Autodesk Inventor part; units mm, degrees
(part 3 of 3)
  arc A561 (-5.9494, 3.2712) -> (-5.9494, -2.9864) centre (0.0316, 0.1424) ccw projected
  arc A562 (-5.9494, 3.2712) -> (-5.9494, -2.9864) centre (0.0316, 0.1424) ccw projected
  arc A563 (-5.9494, 3.2712) -> (-5.9494, -2.9864) centre (0.0316, 0.1424) ccw projected
  arc A564 (-5.9494, 3.2712) -> (-5.9494, -2.9864) centre (0.0316, 0.1424) ccw projected
  arc A565 (-5.9494, 3.2712) -> (-5.9494, -2.9864) centre (0.0316, 0.1424) ccw projected
  arc A566 (-5.9494, 3.2712) -> (-5.9494, -2.9864) centre (0.0316, 0.1424) ccw projected
  circle A567 centre (0.0316, 0.1424) radius 2.5 projected
  circle A568 centre (0.0316, 0.1424) radius 2.5 projected
  circle A569 centre (0.0316, 0.1424) radius 2.5 projected
  circle A570 centre (0.0316, 0.1424) radius 2.5 projected
  circle A571 centre (0.0316, 0.1424) radius 5.5 projected
  circle A572 centre (0.0316, 0.1424) radius 6.75 projected
  arc A573 (3.1605, 6.1234) -> (-3.0972, 6.1234) centre (0.0316, 0.1424) ccw projected
  arc A574 (3.1605, 6.1234) -> (-3.0972, 6.1234) centre (0.0316, 0.1424) ccw projected
  arc A575 (3.1605, 6.1234) -> (-3.0972, 6.1234) centre (0.0316, 0.1424) ccw projected
  arc A576 (3.1605, 6.1234) -> (-3.0972, 6.1234) centre (0.0316, 0.1424) ccw projected
  arc A577 (3.1605, 6.1234) -> (-3.0972, 6.1234) centre (0.0316, 0.1424) ccw projected
  arc A578 (3.1605, 6.1234) -> (-3.0972, 6.1234) centre (0.0316, 0.1424) ccw projected
  arc A579 (6.0127, -2.9864) -> (6.0127, 3.2712) centre (0.0316, 0.1424) ccw projected
  arc A580 (6.0127, -2.9864) -> (6.0127, 3.2712) centre (0.0316, 0.1424) ccw projected
  arc A581 (6.0127, -2.9864) -> (6.0127, 3.2712) centre (0.0316, 0.1424) ccw projected
  arc A582 (6.0127, -2.9864) -> (6.0127, 3.2712) centre (0.0316, 0.1424) ccw projected
  arc A583 (6.0127, -2.9864) -> (6.0127, 3.2712) centre (0.0316, 0.1424) ccw projected
  arc A584 (6.0127, -2.9864) -> (6.0127, 3.2712) centre (0.0316, 0.1424) ccw projected
  line L286 (0.0316, 0.1424) -> (12.7316, 0.1424) projected
  line L287 (0.0316, 0.1424) -> (12.7316, 0.1424) projected
  line L288 (3.1605, 12.915) -> (3.1605, 6.1234) projected
  line L289 (3.1605, 12.915) -> (3.1605, 6.1234) projected
  line L290 (0.0316, 0.1424) -> (0.0316, 12.8424) projected
  line L291 (0.0316, 0.1424) -> (0.0316, 12.8424) projected
  circle A585 centre (8.6605, 19.3778) radius 1.5 projected
  line L292 (6.1605, 19.3778) -> (3.1605, 19.3778) projected
  arc A586 (4.7714, 23.2669) -> (3.1605, 19.3778) centre (8.6605, 19.3778) ccw projected
  arc A587 (4.7714, 23.2669) -> (3.1605, 19.3778) centre (8.6605, 19.3778) ccw projected
  arc A588 (4.7714, 23.2669) -> (3.1605, 19.3778) centre (8.6605, 19.3778) ccw projected
  circle A589 centre (8.6605, 19.3778) radius 2.5 projected
  circle A590 centre (8.6605, 19.3778) radius 2.5 projected
  circle A591 centre (8.6605, 19.3778) radius 3 projected
  arc A592 (3.1605, 19.3778) -> (4.7714, 23.2669) centre (8.6605, 19.3778) ccw projected
  arc A593 (3.1605, 19.3778) -> (4.7714, 23.2669) centre (8.6605, 19.3778) ccw projected
  circle A594 centre (8.6605, 19.3778) radius 5.5 projected
  circle A595 centre (8.6605, 19.3778) radius 5.5 projected
  circle A596 centre (8.6605, 19.3778) radius 5.5 projected
  circle A597 centre (8.6605, 19.3778) radius 5.5 projected
  arc A598 (3.1605, 19.3778) -> (4.7714, 23.2669) centre (8.6605, 19.3778) ccw projected
  line L293 (6.0127, 3.2712) -> (19.2671, 3.2712) projected
  line L294 (6.0127, 3.2712) -> (19.2671, 3.2712) projected
  line L295 (6.0127, 3.2712) -> (19.2671, 3.2712) projected
  line L296 (19.2671, 3.2712) -> (6.0127, 3.2712) projected
  line L297 (6.0127, 3.2712) -> (19.2671, 3.2712) projected
  line L298 (6.0127, 3.2712) -> (19.2671, 3.2712) projected
  line L299 (6.0127, 3.2712) -> (19.2671, 3.2712) projected
  line L300 (22.4784, 40.9739) -> (4.7714, 23.2669) projected
  line L301 (22.4784, 40.9739) -> (4.7714, 23.2669) projected
  line L302 (13.2567, 31.7522) -> (4.7714, 23.2669) projected
  line L303 (13.2567, 31.7522) -> (4.7714, 23.2669) projected
  line L304 (22.4784, 40.9739) -> (13.2567, 31.7522) projected
  line L305 (13.2567, 31.7522) -> (4.7714, 23.2669) projected
  line L306 (22.4784, 40.9739) -> (4.7714, 23.2669) projected
  line L307 (13.2567, 31.7522) -> (4.7714, 23.2669) projected
  circle A599 centre (17.1458, 27.8631) radius 1.5 projected
  circle A600 centre (17.1458, 27.8631) radius 3 projected
  circle A601 centre (17.1458, 27.8631) radius 2.5 projected
  circle A602 centre (17.1458, 27.8631) radius 2.5 projected
  circle A603 centre (17.1458, 27.8631) radius 5.5 projected
  circle A604 centre (17.1458, 27.8631) radius 5.5 projected
  circle A605 centre (17.1458, 27.8631) radius 5.5 projected
  circle A606 centre (17.1458, 27.8631) radius 5.5 projected
  circle A607 centre (17.1458, 27.8631) radius 5.5 projected
  circle A608 centre (17.1458, 27.8631) radius 5.5 projected
  circle A609 centre (17.1458, 27.8631) radius 5.5 projected
  arc A610 (19.2671, 3.2712) -> (23.1562, 4.8822) centre (19.2671, 8.7712) ccw projected
  arc A611 (19.2671, 3.2712) -> (23.1562, 4.8822) centre (19.2671, 8.7712) ccw projected
  arc A612 (19.2671, 3.2712) -> (23.1562, 4.8822) centre (19.2671, 8.7712) ccw projected
  circle A613 centre (19.2671, 8.7712) radius 1.5 projected
  circle A614 centre (19.2671, 8.7712) radius 2.5 projected
  circle A615 centre (19.2671, 8.7712) radius 2.5 projected
  circle A616 centre (19.2671, 8.7712) radius 3 projected
  arc A617 (23.1562, 4.8822) -> (19.2671, 3.2712) centre (19.2671, 8.7712) ccw projected
  arc A618 (23.1562, 4.8822) -> (19.2671, 3.2712) centre (19.2671, 8.7712) ccw projected
  circle A619 centre (19.2671, 8.7712) radius 5.5 projected
  circle A620 centre (19.2671, 8.7712) radius 5.5 projected
  circle A621 centre (19.2671, 8.7712) radius 5.5 projected
  arc A622 (23.1562, 4.8822) -> (19.2671, 3.2712) centre (19.2671, 8.7712) ccw projected
  circle A623 centre (19.2671, 8.7712) radius 5.5 projected
  arc A624 (14.3956, 11.3243) -> (23.1562, 4.8822) centre (19.2671, 8.7712) ccw projected
  line L308 (23.1562, 4.8822) -> (31.6415, 13.3674) projected
  line L309 (23.1562, 4.8822) -> (31.6415, 13.3674) projected
  line L310 (23.1562, 4.8822) -> (31.6415, 13.3674) projected
  line L311 (31.6415, 13.3674) -> (23.1562, 4.8822) projected
  line L312 (22.4784, 40.9739) -> (13.2567, 31.7522) projected
  line L313 (22.4784, 40.9739) -> (13.2567, 31.7522) projected
  line L314 (13.2567, 31.7522) -> (22.4784, 40.9739) projected
  line L315 (33.6153, 29.837) -> (29.7263, 33.7261) projected
  line L316 (29.7263, 33.7261) -> (22.4784, 40.9739) projected
  line L317 (40.8632, 22.5892) -> (22.4784, 40.9739) projected
  line L318 (40.8632, 22.5892) -> (22.4784, 40.9739) projected
  line L319 (40.8632, 22.5892) -> (22.4784, 40.9739) projected
  line L320 (40.8632, 22.5892) -> (22.4784, 40.9739) projected
  line L321 (40.8632, 22.5892) -> (22.4784, 40.9739) projected
  line L322 (40.8632, 22.5892) -> (22.4784, 40.9739) projected
  line L323 (33.6153, 29.837) -> (40.8632, 22.5892) projected
  line L324 (31.6415, 13.3674) -> (40.8632, 22.5892) projected
  circle A625 centre (27.7524, 17.2565) radius 1.5 projected
  circle A626 centre (27.7524, 17.2565) radius 2.5 projected
  circle A627 centre (27.7524, 17.2565) radius 2.5 projected
  circle A628 centre (27.7524, 17.2565) radius 3 projected
  circle A629 centre (27.7524, 17.2565) radius 5.5 projected
  circle A630 centre (27.7524, 17.2565) radius 5.5 projected
  circle A631 centre (27.7524, 17.2565) radius 5.5 projected
  circle A632 centre (27.7524, 17.2565) radius 5.5 projected
  circle A633 centre (27.7524, 17.2565) radius 5.5 projected
  circle A634 centre (27.7524, 17.2565) radius 5.5 projected
  circle A635 centre (27.7524, 17.2565) radius 5.5 projected
  line L325 (23.1562, 4.8822) -> (40.8632, 22.5892) projected
  line L326 (23.1562, 4.8822) -> (40.8632, 22.5892) projected
  line L327 (23.1562, 4.8822) -> (40.8632, 22.5892) projected
  line L328 (31.6415, 13.3674) -> (40.8632, 22.5892) projected
  line L329 (31.6415, 13.3674) -> (40.8632, 22.5892) projected
  line L330 (31.6415, 13.3674) -> (40.8632, 22.5892) projected
  line L331 (-13.1934, -31.4674) -> (-22.4151, -40.6891) projected
  line L332 (-22.4151, -40.6891) -> (-13.1934, -31.4674) projected
  line L333 (-22.4151, -40.6891) -> (-13.1934, -31.4674) projected
  line L334 (-22.4151, -40.6891) -> (-13.1934, -31.4674) projected
  line L335 (-22.4151, -40.6891) -> (-4.7081, -22.9821) projected
  line L336 (-22.4151, -40.6891) -> (-4.7081, -22.9821) projected
  line L337 (-22.4151, -40.6891) -> (-4.7081, -22.9821) projected
  circle A636 centre (-17.0825, -27.5783) radius 1.5 projected
  circle A637 centre (-17.0825, -27.5783) radius 2.5 projected
  circle A638 centre (-17.0825, -27.5783) radius 2.5 projected
  circle A639 centre (-17.0825, -27.5783) radius 5.5 projected
  circle A640 centre (-17.0825, -27.5783) radius 5.5 projected
  circle A641 centre (-17.0825, -27.5783) radius 5.5 projected
  circle A642 centre (-17.0825, -27.5783) radius 5.5 projected
  circle A643 centre (-17.0825, -27.5783) radius 5.5 projected
  circle A644 centre (-17.0825, -27.5783) radius 5.5 projected
  circle A645 centre (-17.0825, -27.5783) radius 5.5 projected
  line L338 (6.1605, -19.0931) -> (3.1605, -19.0931) projected
  arc A646 (3.1605, -19.0931) -> (4.7714, -22.9821) centre (8.6605, -19.0931) ccw projected
  arc A647 (3.1605, -19.0931) -> (4.7714, -22.9821) centre (8.6605, -19.0931) ccw projected
  arc A648 (3.1605, -19.0931) -> (4.7714, -22.9821) centre (8.6605, -19.0931) ccw projected
  line L339 (3.1605, -19.0931) -> (3.1605, -12.6302) projected
  line L340 (3.1605, -19.0931) -> (3.1605, -12.6302) projected
  line L341 (14.3226, -10.9666) -> (14.3956, -11.0396) projected
  circle A649 centre (19.2671, -8.4864) radius 1.5 projected
  circle A650 centre (19.2671, -8.4864) radius 2.5 projected
  circle A651 centre (19.2671, -8.4864) radius 2.5 projected
  circle A652 centre (19.2671, -8.4864) radius 2.5 projected
  circle A653 centre (19.2671, -8.4864) radius 2.5 projected
  arc A654 (23.1562, -4.5974) -> (14.3956, -11.0396) centre (19.2671, -8.4864) ccw projected
  line L342 (17.4993, -10.2542) -> (23.1562, -4.5974) projected
  arc A655 (23.1562, -4.5974) -> (14.3956, -11.0396) centre (19.2671, -8.4864) ccw projected
  line L343 (-5.9494, -2.9864) -> (-19.2038, -2.9864) projected
  line L344 (-5.9494, -2.9864) -> (-19.2038, -2.9864) projected
  line L345 (-5.9494, -2.9864) -> (-19.2038, -2.9864) projected
  line L346 (-5.9494, -2.9864) -> (-19.2038, -2.9864) projected
  line L347 (-5.9494, -2.9864) -> (-19.2038, -2.9864) projected
  line L348 (-5.9494, -2.9864) -> (-19.2038, -2.9864) projected
  line L349 (-19.2038, -2.9864) -> (-5.9494, -2.9864) projected
  arc A656 (4.7714, -22.9821) -> (3.1605, -19.0931) centre (8.6605, -19.0931) ccw projected
  arc A657 (4.7714, -22.9821) -> (3.1605, -19.0931) centre (8.6605, -19.0931) ccw projected
  circle A658 centre (8.6605, -19.0931) radius 5.5 projected
  circle A659 centre (8.6605, -19.0931) radius 5.5 projected
  arc A660 (4.7714, -22.9821) -> (3.1605, -19.0931) centre (8.6605, -19.0931) ccw projected
  circle A661 centre (8.6605, -19.0931) radius 5.5 projected
  circle A662 centre (8.6605, -19.0931) radius 5.5 projected
  circle A663 centre (8.6605, -19.0931) radius 5.5 projected
  circle A664 centre (8.6605, -19.0931) radius 2.5 projected
  circle A665 centre (8.6605, -19.0931) radius 2.5 projected
  circle A666 centre (8.6605, -19.0931) radius 2.5 projected
  circle A667 centre (8.6605, -19.0931) radius 1.5 projected
  line L350 (-23.0929, -4.5974) -> (-40.7999, -22.3044) projected
  circle A668 centre (-27.6891, -16.9717) radius 1.5 projected
  circle A669 centre (-27.6891, -16.9717) radius 2.5 projected
  circle A670 centre (-27.6891, -16.9717) radius 2.5 projected
  line L351 (-23.0929, -4.5974) -> (-40.7999, -22.3044) projected
  line L352 (-23.0929, -4.5974) -> (-40.7999, -22.3044) projected
  line L353 (-31.5782, -13.0826) -> (-40.7999, -22.3044) projected
  circle A671 centre (-27.6891, -16.9717) radius 5.5 projected
  circle A672 centre (-27.6891, -16.9717) radius 5.5 projected
  circle A673 centre (-27.6891, -16.9717) radius 5.5 projected
  circle A674 centre (-27.6891, -16.9717) radius 5.5 projected
  circle A675 centre (-27.6891, -16.9717) radius 5.5 projected
  circle A676 centre (-27.6891, -16.9717) radius 5.5 projected
  circle A677 centre (-27.6891, -16.9717) radius 5.5 projected
  line L354 (-6.9395, -3.6467) -> (-6.2792, -2.9864) projected
  line L355 (0.0316, 0.1424) -> (-12.6684, 0.1424) projected
  line L356 (0.0316, 0.1424) -> (-12.6684, 0.1424) projected
  line L357 (0.0316, 0.1424) -> (0.0316, -12.5576) projected
  line L358 (-23.0929, -4.5974) -> (-31.5782, -13.0826) projected
  line L359 (-23.0929, -4.5974) -> (-31.5782, -13.0826) projected
  line L360 (-23.0929, -4.5974) -> (-31.5782, -13.0826) projected
  arc A678 (-19.2038, -2.9864) -> (-23.0929, -4.5974) centre (-19.2038, -8.4864) ccw projected
  arc A679 (-23.0929, -4.5974) -> (-19.2038, -2.9864) centre (-19.2038, -8.4864) ccw projected
  arc A680 (-19.2038, -2.9864) -> (-23.0929, -4.5974) centre (-19.2038, -8.4864) ccw projected
  arc A681 (-23.0929, -4.5974) -> (-19.2038, -2.9864) centre (-19.2038, -8.4864) ccw projected
  circle A682 centre (-19.2038, -8.4864) radius 5.5 projected
  circle A683 centre (-19.2038, -8.4864) radius 5.5 projected
  arc A684 (-19.2038, -2.9864) -> (-23.0929, -4.5974) centre (-19.2038, -8.4864) ccw projected
  arc A685 (-23.0929, -4.5974) -> (-19.2038, -2.9864) centre (-19.2038, -8.4864) ccw projected
  circle A686 centre (-19.2038, -8.4864) radius 5.5 projected
  line L361 (-31.5782, -13.0826) -> (-23.0929, -4.5974) projected
  circle A687 centre (-19.2038, -8.4864) radius 2.5 projected
  circle A688 centre (-19.2038, -8.4864) radius 2.5 projected
  circle A689 centre (-19.2038, -8.4864) radius 5.5 projected
  arc A690 (-14.3323, -11.0396) -> (-23.0929, -4.5974) centre (-19.2038, -8.4864) ccw projected
  arc A691 (-14.3323, -11.0396) -> (-23.0929, -4.5974) centre (-19.2038, -8.4864) ccw projected
  circle A692 centre (-19.2038, -8.4864) radius 1.5 projected
  arc A693 (-3.0972, -5.8386) -> (3.1605, -5.8386) centre (0.0316, 0.1424) ccw projected
  arc A694 (-3.0972, -5.8386) -> (3.1605, -5.8386) centre (0.0316, 0.1424) ccw projected
  arc A695 (-3.0972, -5.8386) -> (3.1605, -5.8386) centre (0.0316, 0.1424) ccw projected
  arc A696 (-3.0972, -5.8386) -> (3.1605, -5.8386) centre (0.0316, 0.1424) ccw projected
  arc A697 (-3.0972, -5.8386) -> (3.1605, -5.8386) centre (0.0316, 0.1424) ccw projected
  arc A698 (-3.0972, -5.8386) -> (3.1605, -5.8386) centre (0.0316, 0.1424) ccw projected
  line L362 (3.1605, -12.6302) -> (3.1605, -5.8386) projected
  line L363 (3.1605, -12.6302) -> (3.1605, -5.8386) projected
  line L364 (-3.0972, -12.6302) -> (-3.0972, -5.8386) projected
  line L365 (-3.0972, -12.6302) -> (-3.0972, -5.8386) projected
  circle A699 centre (0.0316, -12.5576) radius 2.5 projected
  circle A700 centre (0.0316, -12.5576) radius 2.5 projected
  line L366 (3.1605, -5.8386) -> (3.1605, -19.0931) projected
  line L367 (-3.0972, -19.0931) -> (-3.0972, -5.8386) projected
  line L368 (-3.0972, -19.0931) -> (-3.0972, -5.8386) projected
  line L369 (-3.0972, -19.0931) -> (-3.0972, -5.8386) projected
  line L370 (-3.0972, -19.0931) -> (-3.0972, -5.8386) projected
  line L371 (-3.0972, -19.0931) -> (-3.0972, -5.8386) projected
  line L372 (-3.0972, -19.0931) -> (-3.0972, -5.8386) projected
  line L373 (3.1605, -5.8386) -> (3.1605, -19.0931) projected
  line L374 (3.1605, -5.8386) -> (3.1605, -19.0931) projected
  line L375 (3.1605, -5.8386) -> (3.1605, -19.0931) projected
  line L376 (3.1605, -5.8386) -> (3.1605, -19.0931) projected
  line L377 (3.1605, -5.8386) -> (3.1605, -19.0931) projected
  line L378 (-6.0972, -19.0931) -> (-3.0972, -19.0931) projected
  line L379 (-3.0972, -19.0931) -> (-3.0972, -12.6302) projected
  line L380 (-3.0972, -19.0931) -> (-3.0972, -12.6302) projected
  line L381 (-31.5782, -13.0826) -> (-40.7999, -22.3044) projected
  line L382 (-31.5782, -13.0826) -> (-40.7999, -22.3044) projected
  line L383 (-31.5782, -13.0826) -> (-40.7999, -22.3044) projected
  line L384 (-40.7999, -22.3044) -> (-22.4151, -40.6891) projected
  line L385 (-40.7999, -22.3044) -> (-22.4151, -40.6891) projected
  line L386 (-40.7999, -22.3044) -> (-22.4151, -40.6891) projected
  line L387 (-40.7999, -22.3044) -> (-22.4151, -40.6891) projected
  line L388 (-33.5521, -29.5522) -> (-40.7999, -22.3044) projected
  line L389 (-33.5521, -29.5522) -> (-29.663, -33.4413) projected
  line L390 (-29.663, -33.4413) -> (-22.4151, -40.6891) projected
  line L391 (-40.7999, -22.3044) -> (-22.4151, -40.6891) projected
  line L392 (-40.7999, -22.3044) -> (-22.4151, -40.6891) projected
  arc A701 (-4.7081, -22.9821) -> (-3.0972, -19.0931) centre (-8.5972, -19.0931) ccw projected
  arc A702 (-3.0972, -19.0931) -> (-4.7081, -22.9821) centre (-8.5972, -19.0931) ccw projected
  line L393 (-13.1934, -31.4674) -> (-4.7081, -22.9821) projected
  arc A703 (-4.7081, -22.9821) -> (-3.0972, -19.0931) centre (-8.5972, -19.0931) ccw projected
  line L394 (-13.1934, -31.4674) -> (-4.7081, -22.9821) projected
  arc A704 (-3.0972, -19.0931) -> (-4.7081, -22.9821) centre (-8.5972, -19.0931) ccw projected
  circle A705 centre (-8.5972, -19.0931) radius 5.5 projected
  circle A706 centre (-8.5972, -19.0931) radius 5.5 projected
  circle A707 centre (-8.5972, -19.0931) radius 1.5 projected
  circle A708 centre (-8.5972, -19.0931) radius 2.5 projected
  circle A709 centre (-8.5972, -19.0931) radius 2.5 projected
  circle A710 centre (-8.5972, -19.0931) radius 5.5 projected
  arc A711 (-3.0972, -19.0931) -> (-4.7081, -22.9821) centre (-8.5972, -19.0931) ccw projected
  circle A712 centre (-8.5972, -19.0931) radius 5.5 projected
  arc A713 (-4.7081, -22.9821) -> (-3.0972, -19.0931) centre (-8.5972, -19.0931) ccw projected
  line L395 (-13.1934, -31.4674) -> (-4.7081, -22.9821) projected
  line L396 (-13.1934, -31.4674) -> (-4.7081, -22.9821) projected
  line L397 (12.7316, -10.3076) -> (12.7316, -12.5576) projected
  line L398 (12.7316, -10.3076) -> (12.7316, -12.5576) projected
  line L399 (12.7316, -10.3076) -> (12.7316, -12.5576) projected
  line L400 (12.7316, -12.5576) -> (10.4816, -12.5576) projected
  line L401 (12.7316, -12.5576) -> (10.4816, -12.5576) projected
  line L402 (12.7316, -12.5576) -> (10.4816, -12.5576) projected
  arc A714 (10.4816, -12.5576) -> (11.1407, -14.1486) centre (12.7316, -12.5576) ccw projected
  arc A715 (10.4816, -12.5576) -> (11.1407, -14.1486) centre (12.7316, -12.5576) ccw projected
  arc A716 (10.4816, -12.5576) -> (11.1407, -14.1486) centre (12.7316, -12.5576) ccw projected
  arc A717 (10.5886, -13.2429) -> (11.1407, -14.1486) centre (12.7316, -12.5576) ccw projected
  arc A718 (10.5886, -13.2429) -> (11.1407, -14.1486) centre (12.7316, -12.5576) ccw projected
  arc A719 (23.1562, -4.5974) -> (19.2671, -2.9864) centre (19.2671, -8.4864) ccw projected
  arc A720 (23.1562, -4.5974) -> (19.2671, -2.9864) centre (19.2671, -8.4864) ccw projected
  arc A721 (23.1562, -4.5974) -> (19.2671, -2.9864) centre (19.2671, -8.4864) ccw projected
  arc A722 (23.1562, -4.5974) -> (14.3956, -11.0396) centre (19.2671, -8.4864) ccw projected
  line L403 (15.378, -12.3755) -> (15.9083, -11.8452) projected
  line L404 (15.5548, -12.1988) -> (15.9136, -12.5576) projected
  arc A723 (15.378, -12.3755) -> (15.569, -12.5576) centre (19.2671, -8.4864) ccw projected
  arc A724 (15.378, -12.3755) -> (15.569, -12.5576) centre (19.2671, -8.4864) ccw projected
  arc A725 (19.2671, -2.9864) -> (23.1562, -4.5974) centre (19.2671, -8.4864) ccw projected
  arc A726 (19.2671, -2.9864) -> (23.1562, -4.5974) centre (19.2671, -8.4864) ccw projected
  circle A727 centre (19.2671, -8.4864) radius 5.5 projected
  arc A728 (19.2671, -2.9864) -> (23.1562, -4.5974) centre (19.2671, -8.4864) ccw projected
  circle A729 centre (19.2671, -8.4864) radius 5.5 projected
  circle A730 centre (19.2671, -8.4864) radius 5.5 projected
  circle A731 centre (19.2671, -8.4864) radius 5.5 projected
  line L405 (17.5046, -14.1486) -> (14.3226, -10.9666) projected
  line L406 (24.3936, -20.3305) -> (16.8521, -20.3305) construction
  line L407 (17.5046, -14.1486) -> (26.1667, -22.8107) projected
  line L408 (26.1667, -22.8107) -> (14.3226, -10.9666) projected
  line L409 (14.3226, -10.9666) -> (26.1667, -22.8107) projected
  line L410 (26.1667, -22.8107) -> (14.3226, -10.9666) projected
  arc A732 (14.3226, -17.3306) -> (18.0567, -15.0542) centre (15.9136, -15.7396) ccw projected
  arc A733 (14.3226, -17.3306) -> (17.5046, -14.1486) centre (15.9136, -15.7396) ccw projected
  arc A734 (14.3226, -17.3306) -> (17.5046, -14.1486) centre (15.9136, -15.7396) ccw projected
  line L411 (20.5045, -20.3305) -> (23.3382, -23.1642) projected
  line L412 (20.5045, -20.3305) -> (23.3382, -23.1642) projected
  line L413 (20.5045, -24.2196) -> (13.9798, -17.6948) projected
  line L414 (12.3728, -15.3807) -> (12.5496, -15.204) projected
  line L415 (22.9847, -25.9926) -> (14.3226, -17.3306) projected
  line L416 (11.1407, -14.1486) -> (12.3728, -15.3807) projected
  line L417 (11.1407, -14.1486) -> (14.3226, -17.3306) projected
  line L418 (11.1407, -14.1486) -> (22.9847, -25.9926) projected
  line L419 (11.1407, -14.1486) -> (22.9847, -25.9926) projected
  line L420 (22.9847, -25.9926) -> (11.1407, -14.1486) projected
  line L421 (23.1615, -25.8159) -> (10.5886, -13.2429) projected
  line L422 (23.1615, -25.8159) -> (10.5886, -13.2429) projected
  line L423 (25.9899, -22.9874) -> (13.417, -10.4145) projected
  line L424 (40.8632, -22.3044) -> (23.1562, -4.5974) projected
  line L425 (40.8632, -22.3044) -> (23.1562, -4.5974) projected
  line L426 (31.6415, -13.0826) -> (23.1562, -4.5974) projected
  line L427 (31.6415, -13.0826) -> (23.1562, -4.5974) projected
  line L428 (31.6415, -13.0826) -> (23.1562, -4.5974) projected
  line L429 (31.6415, -13.0826) -> (23.1562, -4.5974) projected
  line L430 (31.6415, -13.0826) -> (23.1562, -4.5974) projected
  arc A735 (31.6415, -13.0826) -> (22.4331, -18.3699) centre (27.7524, -16.9717) ccw projected
  line L431 (22.4331, -18.3699) -> (26.3542, -22.291) projected
  line L432 (40.8632, -22.3044) -> (23.1562, -4.5974) projected
  arc A736 (26.3542, -22.291) -> (31.6415, -13.0826) centre (27.7524, -16.9717) ccw projected
  line L433 (40.8632, -22.3044) -> (31.6415, -13.0826) projected
  line L434 (4.7714, -22.9821) -> (22.4784, -40.6891) projected
  line L435 (22.4784, -40.6891) -> (40.8632, -22.3044) projected
  line L436 (4.7714, -22.9821) -> (22.4784, -40.6891) projected
  line L437 (22.4784, -40.6891) -> (40.8632, -22.3044) projected
  line L438 (22.4784, -40.6891) -> (40.8632, -22.3044) projected
  line L439 (13.2567, -31.4674) -> (22.4784, -40.6891) projected
  arc A737 (13.2567, -31.4674) -> (22.4651, -26.1801) centre (17.1458, -27.5783) ccw projected
  line L440 (22.4651, -26.1801) -> (18.544, -22.259) projected
  arc A738 (18.544, -22.259) -> (13.2567, -31.4674) centre (17.1458, -27.5783) ccw projected
  line L441 (4.7714, -22.9821) -> (13.2567, -31.4674) projected
  line L442 (4.7714, -22.9821) -> (13.2567, -31.4674) projected
  line L443 (4.7714, -22.9821) -> (13.2567, -31.4674) projected
  line L444 (13.2567, -31.4674) -> (4.7714, -22.9821) projected
  line L445 (13.2567, -31.4674) -> (4.7714, -22.9821) projected
  line L446 (4.7714, -22.9821) -> (22.4784, -40.6891) projected
  line L447 (19.2671, -2.9864) -> (6.0127, -2.9864) projected
  line L448 (19.2671, -2.9864) -> (6.0127, -2.9864) projected
  line L449 (19.2671, -2.9864) -> (6.0127, -2.9864) projected
  line L450 (19.2671, -2.9864) -> (6.0127, -2.9864) projected
  line L451 (19.2671, -2.9864) -> (6.0127, -2.9864) projected
  line L452 (19.2671, -2.9864) -> (6.0127, -2.9864) projected
  arc A739 (14.3226, -10.9666) -> (13.417, -10.4145) centre (12.7316, -12.5576) ccw projected
  arc A740 (14.3226, -10.9666) -> (13.417, -10.4145) centre (12.7316, -12.5576) ccw projected
  arc A741 (14.3226, -10.9666) -> (12.7316, -10.3076) centre (12.7316, -12.5576) ccw projected
  arc A742 (14.3226, -10.9666) -> (12.7316, -10.3076) centre (12.7316, -12.5576) ccw projected
  arc A743 (14.3226, -10.9666) -> (12.7316, -10.3076) centre (12.7316, -12.5576) ccw projected
  line L453 (7.0028, -3.6467) -> (6.3425, -2.9864) projected
  line L454 (19.2671, -2.9864) -> (6.0127, -2.9864) projected
  line L455 (19.2671, -2.9864) -> (6.0127, -2.9864) projected
  line L456 (14.3226, -10.9666) -> (7.0028, -3.6467) projected
  line L457 (14.3226, -10.9666) -> (3.9708, -10.9666) construction
  line L458 (25.9899, -22.9874) -> (26.1667, -22.8107) projected
  line L459 (26.1667, -22.8107) -> (25.9899, -22.9874) projected
  line L460 (29.7263, -25.6631) -> (33.6153, -29.5522) projected
  line L461 (22.4784, -40.6891) -> (40.8632, -22.3044) projected
  line L462 (22.4784, -40.6891) -> (40.8632, -22.3044) projected
  line L463 (22.4784, -40.6891) -> (40.8632, -22.3044) projected
  line L464 (33.6153, -29.5522) -> (29.7263, -33.4413) projected
  line L465 (33.6153, -29.5522) -> (29.7263, -33.4413) projected
  line L466 (29.1708, -28.9968) -> (27.2263, -30.9413) projected
  line L467 (27.2263, -30.9413) -> (31.1153, -27.0522) projected
  line L468 (25.9899, -29.7049) -> (25.8372, -29.5522) projected
  line L469 (29.7263, -33.4413) -> (25.9899, -29.7049) projected
  line L470 (23.3382, -23.1642) -> (31.6708, -31.4968) projected
  line L471 (23.1615, -25.8159) -> (22.9847, -25.9926) projected
  line L472 (22.9847, -25.9926) -> (23.1615, -25.8159) projected
  line L473 (22.9847, -25.9926) -> (26.1667, -22.8107) projected
  line L474 (26.1667, -22.8107) -> (22.9847, -25.9926) projected
  circle A744 centre (17.1458, -27.5783) radius 2.5 projected
  circle A745 centre (17.1458, -27.5783) radius 1.5 projected
  circle A746 centre (17.1458, -27.5783) radius 2.5 projected
  line L475 (27.7524, -16.9717) -> (31.6415, -13.0826) projected
  line L476 (18.544, -22.259) -> (22.4651, -26.1801) projected
  line L477 (17.1458, -27.5783) -> (13.2567, -31.4674) projected
  circle A747 centre (17.1458, -27.5783) radius 2.5 projected
  line L478 (17.1458, -27.5783) -> (22.4491, -22.275) projected
  line L479 (22.4651, -26.1801) -> (18.544, -22.259) projected
  line L480 (22.4651, -26.1801) -> (18.544, -22.259) projected
  line L481 (18.544, -22.259) -> (22.4651, -26.1801) projected
  line L482 (18.544, -22.259) -> (22.4651, -26.1801) projected
  circle A748 centre (17.1458, -27.5783) radius 5.5 projected
  arc A749 (18.544, -22.259) -> (22.4651, -26.1801) centre (17.1458, -27.5783) ccw projected
  arc A750 (18.544, -22.259) -> (22.4651, -26.1801) centre (17.1458, -27.5783) ccw projected
  arc A751 (18.544, -22.259) -> (22.4651, -26.1801) centre (17.1458, -27.5783) ccw projected
  circle A752 centre (17.1458, -27.5783) radius 5.5 projected
  arc A753 (18.544, -22.259) -> (13.2567, -31.4674) centre (17.1458, -27.5783) ccw projected
  arc A754 (18.544, -22.259) -> (13.2567, -31.4674) centre (17.1458, -27.5783) ccw projected
  circle A755 centre (17.1458, -27.5783) radius 2.5 projected
  line L483 (13.2567, -31.4674) -> (22.4784, -40.6891) projected
  line L484 (13.2567, -31.4674) -> (22.4784, -40.6891) projected
  line L485 (20.5045, -24.2196) -> (25.8372, -29.5522) projected
  line L486 (21.0349, -31.4674) -> (24.3936, -28.1087) projected
  arc A756 (13.2567, -31.4674) -> (22.4651, -26.1801) centre (17.1458, -27.5783) ccw projected
  line L487 (29.7263, -33.4413) -> (22.4784, -40.6891) projected
  line L488 (29.7263, -33.4413) -> (22.4784, -40.6891) projected
  line L489 (13.2567, -31.4674) -> (22.4784, -40.6891) projected
  line L490 (13.2567, -31.4674) -> (22.4784, -40.6891) projected
  arc A757 (13.2567, -31.4674) -> (22.4651, -26.1801) centre (17.1458, -27.5783) ccw projected
  line L491 (28.2827, -24.2196) -> (31.6415, -20.8608) projected
  line L492 (40.8632, -22.3044) -> (31.6415, -13.0826) projected
  line L493 (40.8632, -22.3044) -> (31.6415, -13.0826) projected
  line L494 (33.6153, -29.5522) -> (40.8632, -22.3044) projected
  line L495 (33.6153, -29.5522) -> (40.8632, -22.3044) projected
  line L496 (31.6415, -13.0826) -> (40.8632, -22.3044) projected
  line L497 (31.6415, -13.0826) -> (40.8632, -22.3044) projected
  arc A758 (31.6415, -13.0826) -> (22.4331, -18.3699) centre (27.7524, -16.9717) ccw projected
  arc A759 (26.3542, -22.291) -> (22.4331, -18.3699) centre (27.7524, -16.9717) ccw projected
  circle A760 centre (27.7524, -16.9717) radius 1.5 projected
  circle A761 centre (27.7524, -16.9717) radius 2.5 projected
  circle A762 centre (27.7524, -16.9717) radius 2.5 projected
  circle A763 centre (27.7524, -16.9717) radius 2.5 projected
  circle A764 centre (27.7524, -16.9717) radius 2.5 projected
  line L498 (23.8633, -20.8608) -> (27.7524, -16.9717) projected
  line L499 (24.3936, -20.3305) -> (29.7263, -25.6631) projected
  arc A765 (31.6415, -13.0826) -> (22.4331, -18.3699) centre (27.7524, -16.9717) ccw projected
  arc A766 (26.3542, -22.291) -> (31.6415, -13.0826) centre (27.7524, -16.9717) ccw projected
  line L500 (24.3936, -20.3305) -> (22.4331, -18.3699) projected
  line L501 (26.3542, -22.291) -> (22.4331, -18.3699) projected
  line L502 (22.4331, -18.3699) -> (26.3542, -22.291) projected
  line L503 (22.4331, -18.3699) -> (26.3542, -22.291) projected
  line L504 (26.3542, -22.291) -> (22.4331, -18.3699) projected
  line L505 (26.3542, -22.291) -> (22.4331, -18.3699) projected
  circle A767 centre (27.7524, -16.9717) radius 5.5 projected
  arc A768 (26.3542, -22.291) -> (22.4331, -18.3699) centre (27.7524, -16.9717) ccw projected
  arc A769 (26.3542, -22.291) -> (22.4331, -18.3699) centre (27.7524, -16.9717) ccw projected
  circle A770 centre (27.7524, -16.9717) radius 5.5 projected
  arc A771 (26.3542, -22.291) -> (31.6415, -13.0826) centre (27.7524, -16.9717) ccw projected
  line L506 (-3.0972, 6.1234) -> (-3.0972, 19.3778) projected
  line L507 (-3.0972, 6.1234) -> (-3.0972, 19.3778) projected
  line L508 (-3.0972, 12.915) -> (-3.0972, 6.1234) projected
  line L509 (-3.0972, 12.915) -> (-3.0972, 6.1234) projected
  line L510 (-3.0972, 6.1234) -> (-3.0972, 19.3778) projected
  line L511 (-3.0972, 6.1234) -> (-3.0972, 19.3778) projected
  line L512 (-3.0972, 6.1234) -> (-3.0972, 19.3778) projected
  line L513 (-3.0972, 6.1234) -> (-3.0972, 19.3778) projected
  arc A772 (-3.0972, 19.3778) -> (-4.7081, 23.2669) centre (-8.5972, 19.3778) ccw projected
  arc A773 (-3.0972, 19.3778) -> (-4.7081, 23.2669) centre (-8.5972, 19.3778) ccw projected
  arc A774 (-3.0972, 19.3778) -> (-4.7081, 23.2669) centre (-8.5972, 19.3778) ccw projected
  circle A775 centre (-8.5972, 19.3778) radius 2.5 projected
  arc A776 (-4.7081, 23.2669) -> (-3.0972, 19.3778) centre (-8.5972, 19.3778) ccw projected
  arc A777 (-4.7081, 23.2669) -> (-3.0972, 19.3778) centre (-8.5972, 19.3778) ccw projected
  circle A778 centre (-8.5972, 19.3778) radius 5.5 projected
  circle A779 centre (-8.5972, 19.3778) radius 5.5 projected
  arc A780 (-4.7081, 23.2669) -> (-3.0972, 19.3778) centre (-8.5972, 19.3778) ccw projected
  circle A781 centre (-8.5972, 19.3778) radius 5.5 projected
  circle A782 centre (-8.5972, 19.3778) radius 5.5 projected
  line L514 (-6.0972, 19.3778) -> (-3.0972, 19.3778) projected
  line L515 (-3.0972, 19.3778) -> (-3.0972, 12.915) projected
  line L516 (-3.0972, 19.3778) -> (-3.0972, 12.915) projected
  circle A783 centre (-17.0825, 27.8631) radius 2.5 projected
  line L517 (-4.7081, 23.2669) -> (-13.1934, 31.7522) projected
  line L518 (-4.7081, 23.2669) -> (-13.1934, 31.7522) projected
  line L519 (-13.1934, 31.7522) -> (-4.7081, 23.2669) projected
  circle A784 centre (-17.0825, 27.8631) radius 1.5 projected
  circle A785 centre (-8.5972, 19.3778) radius 1.5 projected
  circle A786 centre (-8.5972, 19.3778) radius 2.5 projected
  circle A787 centre (-17.0825, 27.8631) radius 2.5 projected
  line L520 (-4.7081, 23.2669) -> (-22.4151, 40.9739) projected
  line L521 (-4.7081, 23.2669) -> (-22.4151, 40.9739) projected
  line L522 (-13.1934, 31.7522) -> (-22.4151, 40.9739) projected
  circle A788 centre (-17.0825, 27.8631) radius 5.5 projected
  line L523 (-13.1934, 31.7522) -> (-22.4151, 40.9739) projected
  line L524 (-4.7081, 23.2669) -> (-13.1934, 31.7522) projected
  line L525 (-13.1934, 31.7522) -> (-22.4151, 40.9739) projected
  line L526 (-4.7081, 23.2669) -> (-22.4151, 40.9739) projected
  circle A789 centre (-17.0825, 27.8631) radius 5.5 projected
  circle A790 centre (-17.0825, 27.8631) radius 5.5 projected
  circle A791 centre (-17.0825, 27.8631) radius 5.5 projected
  circle A792 centre (-17.0825, 27.8631) radius 5.5 projected
  circle A793 centre (-17.0825, 27.8631) radius 5.5 projected
  circle A794 centre (-17.0825, 27.8631) radius 5.5 projected
  arc A795 (-23.0929, 4.8822) -> (-19.2038, 3.2712) centre (-19.2038, 8.7712) ccw projected
  line L527 (-19.2038, 3.2712) -> (-5.9494, 3.2712) projected
  line L528 (-6.9395, 3.9315) -> (-6.2792, 3.2712) projected
  circle A796 centre (-19.2038, 8.7712) radius 2.5 projected
  arc A797 (-19.2038, 3.2712) -> (-23.0929, 4.8822) centre (-19.2038, 8.7712) ccw projected
  arc A798 (-19.2038, 3.2712) -> (-23.0929, 4.8822) centre (-19.2038, 8.7712) ccw projected
  arc A799 (-19.2038, 3.2712) -> (-23.0929, 4.8822) centre (-19.2038, 8.7712) ccw projected
  arc A800 (-23.0929, 4.8822) -> (-14.3323, 11.3243) centre (-19.2038, 8.7712) ccw projected
  arc A801 (-23.0929, 4.8822) -> (-19.2038, 3.2712) centre (-19.2038, 8.7712) ccw projected
  line L529 (-19.2038, 3.2712) -> (-5.9494, 3.2712) projected
  line L530 (-19.2038, 3.2712) -> (-5.9494, 3.2712) projected
  line L531 (-19.2038, 3.2712) -> (-5.9494, 3.2712) projected
  line L532 (-19.2038, 3.2712) -> (-5.9494, 3.2712) projected
  line L533 (-19.2038, 3.2712) -> (-5.9494, 3.2712) projected
  line L534 (-19.2038, 3.2712) -> (-5.9494, 3.2712) projected
  circle A802 centre (-19.2038, 8.7712) radius 5.5 projected
  circle A803 centre (-19.2038, 8.7712) radius 5.5 projected
  circle A804 centre (-19.2038, 8.7712) radius 5.5 projected
  arc A805 (-23.0929, 4.8822) -> (-19.2038, 3.2712) centre (-19.2038, 8.7712) ccw projected
  circle A806 centre (-19.2038, 8.7712) radius 1.5 projected
  circle A807 centre (-19.2038, 8.7712) radius 2.5 projected
  arc A808 (-23.0929, 4.8822) -> (-14.3323, 11.3243) centre (-19.2038, 8.7712) ccw projected
  circle A809 centre (-19.2038, 8.7712) radius 5.5 projected
  line L535 (-29.663, 33.7261) -> (-22.4151, 40.9739) projected
  line L536 (-13.1934, 31.7522) -> (-22.4151, 40.9739) projected
  line L537 (-40.7999, 22.5892) -> (-23.0929, 4.8822) projected
  line L538 (-31.5782, 13.3674) -> (-23.0929, 4.8822) projected
  line L539 (-40.7999, 22.5892) -> (-23.0929, 4.8822) projected
  line L540 (-40.7999, 22.5892) -> (-23.0929, 4.8822) projected
  circle A810 centre (-27.6891, 17.2565) radius 5.5 projected
  circle A811 centre (-27.6891, 17.2565) radius 5.5 projected
  circle A812 centre (-27.6891, 17.2565) radius 5.5 projected
  circle A813 centre (-27.6891, 17.2565) radius 5.5 projected
  circle A814 centre (-27.6891, 17.2565) radius 5.5 projected
  circle A815 centre (-27.6891, 17.2565) radius 5.5 projected
  circle A816 centre (-27.6891, 17.2565) radius 5.5 projected
  circle A817 centre (-27.6891, 17.2565) radius 2.5 projected
  circle A818 centre (-27.6891, 17.2565) radius 2.5 projected
  line L541 (-31.5782, 13.3674) -> (-23.0929, 4.8822) projected
  line L542 (-31.5782, 13.3674) -> (-23.0929, 4.8822) projected
  circle A819 centre (-27.8428, 17.2565) radius 1.5 projected
  line L543 (-22.4151, 40.9739) -> (-40.7999, 22.5892) projected
  line L544 (-22.4151, 40.9739) -> (-40.7999, 22.5892) projected
  line L545 (-22.4151, 40.9739) -> (-40.7999, 22.5892) projected
  line L546 (-22.4151, 40.9739) -> (-40.7999, 22.5892) projected
  line L547 (-33.5521, 29.837) -> (-40.7999, 22.5892) projected
  line L548 (-22.4151, 40.9739) -> (-40.7999, 22.5892) projected
  line L549 (-22.4151, 40.9739) -> (-40.7999, 22.5892) projected
  line L550 (-33.5521, 29.837) -> (-29.663, 33.7261) projected
  line L551 (-31.5782, 13.3674) -> (-40.7999, 22.5892) projected
  line L552 (-40.7999, 22.5892) -> (-31.5782, 13.3674) projected
  line L553 (-40.7999, 22.5892) -> (-31.5782, 13.3674) projected
  line L554 (-40.7999, 22.5892) -> (-31.5782, 13.3674) projected
  line L555 (-31.5782, 13.3674) -> (-23.0929, 4.8822) projected
  line L556 (0.0316, 0.1424) -> (-2.7968, 0.1424)
  line L557 (0.0316, 0.1424) -> (0.0316, 3.1476)
  line L558 (-27.6891, -16.9717) -> (-29.8418, -19.1245)
  line L559 (-27.6891, -24.7499) -> (-24.8607, -27.5783)
  line L560 (-17.0825, -27.5783) -> (-19.2352, -29.7311)
  line L561 (-27.6891, -16.9717) -> (-19.2038, -8.4864)
  line L562 (-27.6891, -16.9717) -> (-25.5996, -19.0612)
  line L563 (-23.8, -20.8608) -> (-27.6891, -24.7499)
  line L564 (-20.9716, -23.6892) -> (-24.8607, -27.5783)
  line L565 (-23.8, -20.8608) -> (-15.3147, -12.3755)
  line L566 (-20.9716, -23.6892) -> (-12.4863, -15.204)
  line L567 (-15.3147, -12.3755) -> (-10.0114, -7.0722)
  line L568 (-10.0114, -7.0722) -> (-7.183, -9.9007)
  line L569 (-7.183, -9.9007) -> (-12.4863, -15.204)
  line L570 (27.7524, -24.7499) -> (24.9239, -27.5783)
  line L571 (23.8633, -20.8608) -> (27.7524, -24.7499)
  line L572 (21.0349, -23.6892) -> (24.9239, -27.5783)
  line L573 (23.8633, -20.8608) -> (15.378, -12.3755)
  line L574 (21.0349, -23.6892) -> (12.5496, -15.204)
  line L575 (15.378, -12.3755) -> (10.0747, -7.0722)
  line L576 (10.0747, -7.0722) -> (7.2463, -9.9007)
  line L577 (7.2463, -9.9007) -> (12.5496, -15.204)
  line L578 (-27.6891, 25.0347) -> (-24.8607, 27.8631)
  line L579 (-23.8, 21.1456) -> (-27.6891, 25.0347)
  line L580 (-20.9716, 23.974) -> (-24.8607, 27.8631)
  line L581 (-23.8, 21.1456) -> (-15.3147, 12.6603)
  line L582 (-20.9716, 23.974) -> (-12.4863, 15.4888)
  line L583 (-15.3147, 12.6603) -> (-10.0114, 7.357)
  line L584 (-10.0114, 7.357) -> (-7.183, 10.1855)
  line L585 (-7.183, 10.1855) -> (-12.4863, 15.4888)
  line L586 (23.8633, 21.1456) -> (15.378, 12.6603)
  line L587 (23.8633, 21.1456) -> (27.7524, 25.0347)
  line L588 (27.7524, 25.0347) -> (24.9239, 27.8631)
  line L589 (21.0349, 23.974) -> (24.9239, 27.8631)
  line L590 (21.0349, 23.974) -> (12.5496, 15.4888)
  line L591 (7.2463, 10.1855) -> (12.5496, 15.4888)
  line L592 (15.378, 12.6603) -> (10.0747, 7.357)
  line L593 (10.0747, 7.357) -> (7.2463, 10.1855)
  point P0 (17.5046, -17.3306)
  point P1 (12.0192, -15.7343)
  point P2 (20.2447, -16.8886)
  point P3 (4.7714, 23.2669)
  point P4 (-4.7081, -22.9821)
  point P5 (-3.9075, -10.9666)
  point P6 (-4.7081, 23.2669)
  point P7 (3.9708, 11.2514)
  point P8 (-3.9075, 11.2514)
  point P9 (25.9899, 23.2722)
  point P10 (25.9899, 23.2722)
  point P11 (17.5046, 14.4334)
  point P12 (-17.4413, 14.4334)
  point P13 (-25.9266, 23.2722)
  point P14 (-25.9266, 23.2722)
  point P15 (23.3382, 23.449)
  point P16 (25.9899, 23.2722)
  point P17 (11.1407, 14.4334)
  point P18 (17.5046, 14.4334)
  point P19 (14.3226, 17.6154)
  point P20 (-25.9266, -22.9874)
  point P21 (-17.4413, -14.1486)
  point P22 (15.9136, -15.7396)
  point P23 (11.1407, -14.1486)
  point P24 (17.5046, -17.3306)
  point P25 (17.5046, -14.1486)
  point P26 (14.3226, -17.3306)
  point P27 (10.4816, -12.5576)
  point P28 (10.4816, -12.5576)
  point P29 (12.7316, -12.5576)
  point P30 (12.7316, -10.3076)
  point P31 (12.7316, -10.3076)
  point P32 (12.7316, -12.5576)
  point P33 (10.4816, -12.5576)
  point P34 (10.4816, -12.5576)
  point P35 (14.3226, -17.3306)
  point P36 (17.5046, -14.1486)
  point P37 (17.5046, -17.3306)
  point P38 (11.1407, -14.1486)
  point P39 (15.9136, -15.7396)
  point P40 (-17.4413, -14.1486)
  point P41 (-25.9266, -22.9874)
  point P42 (14.3226, 17.6154)
  point P43 (17.5046, 14.4334)
  point P44 (11.1407, 14.4334)
  point P45 (25.9899, 23.2722)
  point P46 (23.3382, 23.449)
  point P47 (-25.9266, 23.2722)
  point P48 (-25.9266, 23.2722)
  point P49 (-17.4413, 14.4334)
  point P50 (17.5046, 14.4334)
  point P51 (25.9899, 23.2722)
  point P52 (25.9899, 23.2722)
  point P53 (-3.9075, -10.9666)
  point P54 (-4.7081, -22.9821)
  point P55 (4.7714, 23.2669)
  point P56 (-4.7081, 23.2669)
  point P57 (-3.9075, 11.2514)
  point P58 (3.9708, 11.2514)
  point P59 (12.0192, -15.7343)
  point P60 (20.2447, -16.8886)
  point P61 (17.5046, -17.3306)
  dimension "d49" = 7.5
  constraints: 76 end point, 17 point on line, 16 symmetric about line, 14 coincident, 13 vertical, 8 horizontal, 5 collinear, 5 horizontal alignment, 5 perpendicular, 4 tangent, 2 point on circle, 2 vertical alignment, 1 parallel, 721 other
  measures "d49" distance of L565.end L567.end
body "Solid1"
